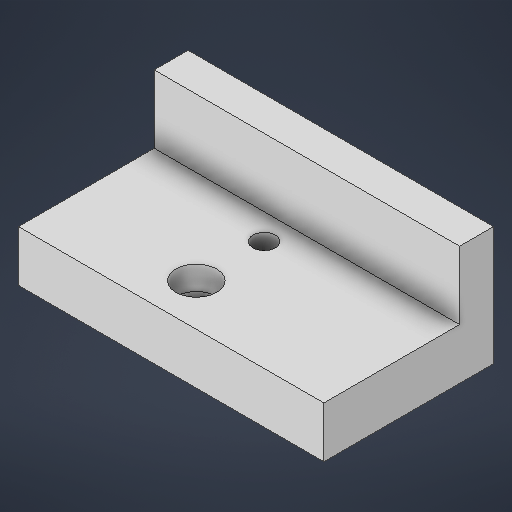
# Autodesk Inventor part: Mount for Slit VA100CP
Saved by Autodesk Inventor 2026 (Build 300175000, 175)
## iProperties
Created: 2026-02-04
Part Number: Mount for Slit VA100CP
Material: Generic
Document SubType Name: Modeling
Designer: FiolkaLab
Density: 1 g/cm^3
Appearance: Default
Author: FiolkaLab
Autodesk Inventor part; units mm, degrees
ref_plane "YZ Plane" through (0, 0, 0) normal (1, 0, 0) x (0, 1, 0)
ref_plane "XZ Plane" through (0, 0, 0) normal (0, 1, 0) x (-1, 0, 0)
ref_plane "XY Plane" through (0, 0, 0) normal (0, 0, 1) x (1, 0, 0)
sketch "Sketch1" plane through (0, 0, 0) normal (0, 1, 0) x (-1, 0, 0)
  line L0 (15.875, -28.575) -> (-15.875, -28.575)
  line L1 (-15.875, -28.575) -> (-15.875, 28.575)
  line L2 (-15.875, 28.575) -> (15.875, 28.575)
  line L3 (15.875, 28.575) -> (15.875, -28.575)
  line L4 (15.875, -28.575) -> (-15.875, 28.575) construction
  line L5 (-15.875, -28.575) -> (15.875, 28.575) construction
  point P0 (0, 0)
  dimension "d0" = 31.75
  dimension "d1" = 57.15
  constraints: 12 end point, 2 midpoint, 2 parallel, 1 horizontal, 1 perpendicular
  measures "d0" distance of L1.end L2.end
  measures "d1" distance of L0.end L1.end
extrude "Extrusion1" add sketch "Sketch1" along normal blind 9.525
sketch "Sketch2" plane through (0, 9.525, 0) normal (0, 1, 0) x (1, 0, 0)
  line L0 (15.875, -28.575) -> (15.875, 28.575) projected
  line L1 (-15.875, -28.575) -> (15.875, -28.575) projected
  line L2 (15.875, 28.575) -> (9.525, 28.575)
  line L3 (9.525, 28.575) -> (9.525, -28.575)
  line L4 (9.525, -28.575) -> (15.875, -28.575)
  line L5 (15.875, -28.575) -> (15.875, 28.575)
  point P0 (0, 0)
  dimension "d4" = 6.35
  constraints: 8 end point, 2 parallel, 1 horizontal, 1 perpendicular, 1 point on line
  measures "d4" distance of L4.end L3.end
extrude "Extrusion2" add sketch "Sketch2" along normal blind 12.7
sketch "Sketch3" plane through (0, 0, 0) normal (0, -1, 0) x (1, 0, 0)
  line L0 (-15.875, 28.575) -> (9.525, 28.575) projected
  point P0 (0, 0)
  point P1 (4.699, -3.175)
  dimension "d14" = 4.826
  dimension "d15" = 31.75
  measures "d14" horizontal distance of L0.end point (4.699, -3.175)
  measures "d15" distance from line of L0 point (4.699, -3.175)
hole "Hole1" at (4.699, 0, -3.175) direction (0, 1, 0) diameter 4.2 end through all counterbore diameter 7.62 counterbore depth 5.08
sketch "Sketch5" plane through (0, 9.525, 0) normal (0, 1, 0) x (1, 0, 0)
  line L0 (9.525, 28.575) -> (-15.875, 28.575) projected
  circle A0 centre (4.699, 3.175) radius 3.81 projected
  line L1 (-15.875, -28.575) -> (9.525, -28.575) projected
  point P0 (0, 0)
  point P1 (-8.001, 3.175)
  dimension "d33" = 12.7
  dimension "d40" = 31.75
  measures "d33" distance of A0.centre point (-8.001, 3.175)
  measures "d40" distance from line of L1 point (-8.001, 3.175)
hole "Hole3" at (-8.001, 9.525, -3.175) direction (0, -1, 0) diameter 4.699 end through all counterbore diameter 7.62 counterbore depth 4.445
sketch "Sketch6" plane through (0, 0, 0) normal (0, -1, 0) x (1, 0, 0)
  circle A0 centre (-8.001, -8.179) radius 1.0125
  circle A1 centre (-8.001, 1.829) radius 1.0125
  circle A2 centre (-8.001, -3.175) radius 2.3495 projected
  point P0 (0, 0)
  dimension "d34" = 2.025
  dimension "d35" = 2.025
  dimension "d36" = 5.004
  dimension "d37" = 5.004
  constraints: 2 centre point
  measures "d34" diameter of A0
  measures "d35" diameter of A1
  measures "d36" distance of A2.centre A0.centre
  measures "d37" distance of A2.centre A1.centre
extrude "Extrusion3" cut sketch "Sketch6" against normal blind 4.826 contours A0 | A1
body "Solid1"
